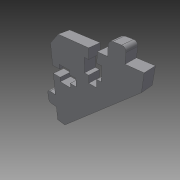
# Autodesk Inventor part: x_carryage_brace_top
Saved by Autodesk Inventor 2014 (Build 180170000, 170)
## iProperties
Created: 2014-03-27
Part Number: x_carryage_brace_top
Material: Plywood, Finish
Document SubType Name: Modeling
Designer: buben
Density: 0.552 g/cm^3
Appearance: Plywood - New
Author: buben
Autodesk Inventor part; units mm, degrees
ref_plane "YZ Plane" through (0, 0, 0) normal (1, 0, 0) x (0, 1, 0)
ref_plane "XZ Plane" through (0, 0, 0) normal (0, 1, 0) x (-1, 0, 0)
ref_plane "XY Plane" through (0, 0, 0) normal (0, 0, 1) x (1, 0, 0)
sketch "Sketch1" plane through (0, 0, 0) normal (0, 1, 0) x (-1, 0, 0)
  line L0 (0, -51.7) -> (0, 0)
  line L1 (0, 0) -> (-50, 0)
  line L2 (-50, 0) -> (-50, -8)
  line L3 (-50, -8) -> (-6, -51.7)
  line L4 (-6, -51.7) -> (0, -51.7)
  dimension "d0" = 51.7
  dimension "d1" = 50
  dimension "d2" = 8
  dimension "d3" = 6
  constraints: 10 end point, 2 parallel, 1 perpendicular, 1 vertical
  measures "d0" distance of L0.start L0.end
  measures "d1" distance of L0.end L1.end
  measures "d2" distance of L1.end L2.end
  measures "d3" distance of L3.end L0.start
extrude "Extrusion1" add sketch "Sketch1" along normal blind 6.5
sketch "Sketch2" plane through (0, 6.5, 0) normal (0, 1, 0) x (1, 0, 0)
  line L0 (0, 0) -> (50, 0) projected
  line L1 (50, 0) -> (50, 8) projected
  line L2 (34, 0) -> (42, 0)
  line L3 (42, 0) -> (42, -4.5)
  line L4 (40, -6.5) -> (36, -6.5)
  line L5 (34, -4.5) -> (34, 0)
  arc A0 (34, -4.5) -> (36, -6.5) centre (36, -4.5) ccw
  arc A1 (40, -6.5) -> (42, -4.5) centre (40, -4.5) ccw
  dimension "d6" = 2
  dimension "d7" = 8
  dimension "d8" = 6.5
  dimension "d9" = 8
  constraints: 8 end point, 4 point on circle, 4 tangent, 2 centre point, 2 parallel, 1 equal radius, 1 horizontal, 1 perpendicular, 1 point on line
  measures "d6" radius of A0
  measures "d7" distance between parallel lines of L3 L5
  measures "d8" distance between parallel lines of L0 L4
  measures "d9" distance between parallel lines of L1 L3
extrude "Extrusion2" add sketch "Sketch2" against normal blind 6.5
sketch "Sketch3" plane through (0, 6.5, 0) normal (0, 1, 0) x (1, 0, 0)
  line L0 (0, 0) -> (34, 0) projected
  line L1 (34, 0) -> (34, -4.5) projected
  line L2 (24.25, 16.3) -> (28.75, 16.3)
  line L3 (28.75, 0) -> (24.25, 0)
  line L4 (31.25, 12.3) -> (31.25, 5)
  line L5 (21.75, 5) -> (21.75, 12.3)
  line L6 (21.75, 12.3) -> (24.25, 12.3)
  line L7 (28.75, 12.3) -> (31.25, 12.3)
  line L8 (24.25, 0) -> (24.25, 5)
  line L9 (24.25, 12.3) -> (24.25, 16.3)
  line L10 (31.25, 5) -> (28.75, 5)
  line L11 (24.25, 5) -> (21.75, 5)
  line L12 (28.75, 16.3) -> (28.75, 12.3)
  line L13 (28.75, 5) -> (28.75, 0)
  point P0 (26.5, 16.3)
  dimension "d12" = 4.5
  dimension "d13" = 5
  dimension "d14" = 7.3
  dimension "d15" = 4
  dimension "d16" = 2.5
  dimension "d17" = 7.5
  constraints: 24 end point, 10 parallel, 6 collinear, 4 perpendicular, 3 horizontal, 1 midpoint
  measures "d12" distance of L2.start L2.end
  measures "d13" distance of L10.end L3.start
  measures "d14" distance of L4.start L4.end
  measures "d15" distance of L2.end L7.start
  measures "d16" distance of L7.start L4.start
  measures "d17" distance from line of L1 point (26.5, 16.3)
extrude "Extrusion3" cut sketch "Sketch3" against normal through all
sketch "Sketch4" plane through (0, 6.5, 0) normal (0, 1, 0) x (1, 0, 0)
  line L0 (0, 51.7) -> (0, 0) projected
  line L1 (0, 0) -> (24.25, 0) projected
  line L2 (16.3, 22) -> (16.3, 17.5)
  line L3 (0, 17.5) -> (0, 22)
  line L4 (5, 24.5) -> (12.3, 24.5)
  line L5 (12.3, 15) -> (5, 15)
  line L6 (0, 22) -> (5, 22)
  line L7 (12.3, 22) -> (16.3, 22)
  line L8 (16.3, 17.5) -> (12.3, 17.5)
  line L9 (5, 17.5) -> (0, 17.5)
  line L10 (5, 15) -> (5, 17.5)
  line L11 (5, 22) -> (5, 24.5)
  line L12 (12.3, 24.5) -> (12.3, 22)
  line L13 (12.3, 17.5) -> (12.3, 15)
  point P0 (16.3, 19.75)
  dimension "d20" = 4.5
  dimension "d21" = 5
  dimension "d22" = 4
  dimension "d23" = 7.3
  dimension "d24" = 19.75
  dimension "d25" = 2.5
  constraints: 24 end point, 10 parallel, 6 collinear, 4 perpendicular, 3 horizontal, 1 midpoint
  measures "d20" distance of L2.start L2.end
  measures "d21" distance of L9.start L3.start
  measures "d22" distance of L2.end L8.end
  measures "d23" distance of L5.start L5.end
  measures "d24" distance from line of L1 point (16.3, 19.75)
  measures "d25" distance of L4.end L7.start
extrude "Extrusion4" cut sketch "Sketch4" against normal through all
sketch "Sketch5" plane through (0, 6.5, 0) normal (0, 1, 0) x (1, 0, 0)
  line L0 (16.3, 22) -> (16.3, 17.5) projected
  line L1 (0, 51.7) -> (0, 22) projected
  line L2 (0, 42.75) -> (-4.5, 42.75)
  line L3 (-6.5, 40.75) -> (-6.5, 36.75)
  line L4 (-4.5, 34.75) -> (0, 34.75)
  line L5 (0, 34.75) -> (0, 42.75)
  arc A0 (-4.5, 42.75) -> (-6.5, 40.75) centre (-4.5, 40.75) ccw
  arc A1 (-6.5, 36.75) -> (-4.5, 34.75) centre (-4.5, 36.75) ccw
  point P0 (16.3, 19.75)
  dimension "d28" = 2
  dimension "d29" = 8
  dimension "d30" = 6.5
  dimension "d31" = 15
  constraints: 8 end point, 4 point on circle, 4 tangent, 2 centre point, 2 parallel, 1 equal radius, 1 horizontal, 1 midpoint, 1 perpendicular, 1 point on line
  measures "d28" radius of A0
  measures "d29" distance between parallel lines of L2 L4
  measures "d30" distance between parallel lines of L5 L3
  measures "d31" distance from line of point (16.3, 19.75) L4
extrude "Extrusion5" add sketch "Sketch5" against normal blind 6.5
chamfer "Chamfer1" distance 6 angle 45 1 edges at (0, 3.25, 0)
body "Solid1"
